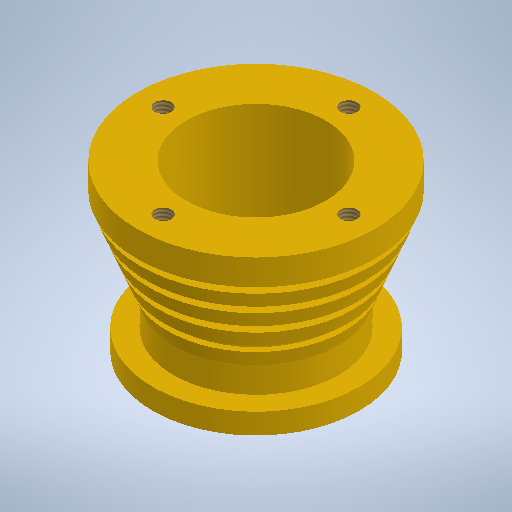
# Autodesk Inventor part: gehaeuse
Saved by Autodesk Inventor 2025 (Build 290162010, 162A)
## iProperties
Created: 2024-07-15
Part Number: gehaeuse
Material: Blei
Document SubType Name: Modeling
Designer: ffogue
Density: 11.34 g/cm^3
Appearance: Gold
Author: ffogue
Autodesk Inventor part; units mm, degrees
note: some values were not read from the file. Chosen so that the rebuilt part matches the saved one: direction of "Bohrung1"; direction of "Bohrung2".
ref_plane "YZ Plane" through (0, 0, 0) normal (1, 0, 0) x (0, 1, 0)
ref_plane "XZ Plane" through (0, 0, 0) normal (0, 1, 0) x (-1, 0, 0)
ref_plane "XY Plane" through (0, 0, 0) normal (0, 0, 1) x (1, 0, 0)
sketch "Skizze1" plane through (0, 0, 0) normal (0, 1, 0) x (-1, 0, 0)
  line L0 (0, 0) -> (0, 32)
  line L1 (0, 32) -> (-23, 32)
  line L2 (-23, 32) -> (-23, 27)
  line L3 (-16, 9) -> (-16, 4)
  line L4 (-16, 4) -> (-20, 4)
  line L5 (-20, 4) -> (-20, 0)
  line L6 (-20, 0) -> (0, 0)
  line L7 (-23, 27) -> (-16, 27)
  line L8 (-16, 27) -> (-16, 25.5)
  line L9 (-16, 25.5) -> (-22.4167, 25.5)
  line L10 (-21.25, 22.5) -> (-16, 22.5)
  line L11 (-16, 22.5) -> (-16, 21)
  line L12 (-16, 21) -> (-20.6667, 21)
  line L13 (-19.5, 18) -> (-16, 18)
  line L14 (-16, 18) -> (-16, 16.5)
  line L15 (-16, 16.5) -> (-18.9167, 16.5)
  line L16 (-17.75, 13.5) -> (-16, 13.5)
  line L17 (-16, 13.5) -> (-16, 12)
  line L18 (-16, 12) -> (-17.1667, 12)
  line L19 (-16, 9) -> (-17.1667, 12)
  line L20 (-17.75, 13.5) -> (-18.9167, 16.5)
  line L21 (-19.5, 18) -> (-20.6667, 21)
  line L22 (-21.25, 22.5) -> (-22.4167, 25.5)
  point P0 (-17.75, 18)
  point P1 (-17.4583, 16.5)
  point P2 (-16.5833, 12)
  point P3 (-16.875, 13.5)
  dimension "d18" = 32
  dimension "d21" = 4
  dimension "d26" = 46
  dimension "d27" = 40
  dimension "d28" = 32
  dimension "d29" = 18
  dimension "d30" = 5
  dimension "d34" = 5
  dimension "d35" = 1.5
  dimension "d36" = 1.5
  dimension "d37" = 1.5
  dimension "d38" = 1.5
  dimension "d42" = 3
  dimension "d43" = 3
  dimension "d44" = 3
  constraints: 46 end point, 9 perpendicular, 6 point on line, 4 midpoint, 4 parallel, 2 horizontal, 1 vertical, 1 vertical alignment
  measures "d18" distance of L0.start L0.end
  measures "d21" distance of L4.end L5.end
  measures "d26" diameter of L2 L0
  measures "d27" diameter of L5 L0
  measures "d28" diameter of L3 L0
  measures "d29" vertical distance of L3.start L2.end
  measures "d30" distance of L1.end L2.end
  measures "d34" distance of L3.end L3.start
  measures "d35" distance between parallel lines of L9 L7
  measures "d36" distance between parallel lines of L12 L10
  measures "d37" distance between parallel lines of L15 L13
  measures "d38" vertical distance of point (-16.583, 12) point (-16.875, 13.5)
  measures "d42" distance between parallel lines of L10 L9
  measures "d43" distance between parallel lines of L13 L12
  measures "d44" distance between parallel lines of L16 L15
revolve "Umdrehung1" add sketch "Skizze1" angle 360 about axis through (0, 0, 0) along (0, 0, 1)
sketch "Skizze2" plane through (0, 0, 32) normal (0, 0, 1) x (1, 0, 0)
  circle A0 centre (0, 0) radius 18 construction
  point P0 (0, -18)
  point P1 (0, 18)
  point P2 (-18, 0)
  point P3 (18, 0)
  dimension "d46" = 36
  constraints: 4 point on circle, 2 horizontal alignment, 2 vertical alignment, 1 centre point, 1 coincident
  measures "d46" diameter of A0
hole "Bohrung1" at (0, -18, 32) at (0, 18, 32) at (-18, 0, 32) at (18, 0, 32) direction (0, 0, -1) diameter 3.242 depth 9.5 thread size "M4x0.7" class "6H" standard "ISO Metric profile"
sketch "Skizze3" plane through (0, 0, 32) normal (0, 0, 1) x (1, 0, 0)
  circle A0 centre (0, 0) radius 23 projected
  constraints: 1 coincident
hole "Bohrung2" at (0, 0, 32) direction (0, 0, -1) diameter 27 depth 32
equation "\"d36\" = d35"
equation "\"d37\" = d35"
equation "\"d38\" = d37"
